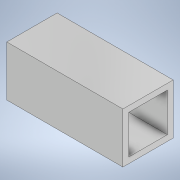
# Autodesk Inventor part: Aluminum box 2x2x6 .3 thickness
Saved by Autodesk Inventor 2021 (Build 250183000, 183)
## iProperties
Created: 2021-03-08
Part Number: Aluminum box 2x2x6 .3 thickness
Material: Generic
Document SubType Name: Modeling
Designer: david
Density: 1 g/cm^3
Appearance: Aluminum - Polished
Author: david
Autodesk Inventor part; units mm, degrees
ref_plane "YZ Plane" through (0, 0, 0) normal (1, 0, 0) x (0, 1, 0)
ref_plane "XZ Plane" through (0, 0, 0) normal (0, 1, 0) x (-1, 0, 0)
ref_plane "XY Plane" through (0, 0, 0) normal (0, 0, 1) x (1, 0, 0)
sketch "Sketch1" plane through (0, 0, 0) normal (1, 0, 0) x (0, 1, 0)
  line L0 (62.1244, -15.24) -> (11.3244, -15.24)
  line L1 (11.3244, -15.24) -> (11.3244, -66.04)
  line L2 (11.3244, -66.04) -> (62.1244, -66.04)
  line L3 (62.1244, -66.04) -> (62.1244, -15.24)
  line L4 (69.7444, -7.62) -> (3.7044, -7.62)
  line L5 (3.7044, -7.62) -> (3.7044, -73.66)
  line L6 (3.7044, -73.66) -> (69.7444, -73.66)
  line L7 (69.7444, -73.66) -> (69.7444, -7.62)
  point P0 (0, 0)
  dimension "d0" = 50.8
  dimension "d1" = 50.8
  dimension "d2" = 7.62
  constraints: 16 end point, 4 parallel, 2 perpendicular, 1 horizontal, 3 other
  measures "d0" distance of L2.end L0.start
  measures "d1" distance of L0.start L0.end
  measures "d2" distance between parallel lines of L3 L7
extrude "Extrusion1" add sketch "Sketch1" along normal blind 152.4
body "Solid1"
